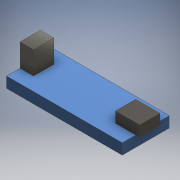
# Autodesk Inventor part: Arduino Nano
Saved by Autodesk Inventor 2016 (Build 200138000, 138)
## iProperties
Created: 2016-05-01
Part Number: Arduino Nano
Material: Generic
Document SubType Name: Modeling
Designer: Owner
Density: 1 g/cm^3
Appearance: Default
Author: Owner
Autodesk Inventor part; units mm, degrees
ref_plane "YZ Plane" through (0, 0, 0) normal (1, 0, 0) x (0, 1, 0)
ref_plane "XZ Plane" through (0, 0, 0) normal (0, 1, 0) x (-1, 0, 0)
ref_plane "XY Plane" through (0, 0, 0) normal (0, 0, 1) x (1, 0, 0)
sketch "Sketch1" plane through (0, 0, 0) normal (0, 0, 1) x (1, 0, 0)
  line L0 (0, 0) -> (43, 0)
  line L1 (43, 0) -> (43, 17.5)
  line L2 (43, 17.5) -> (0, 17.5)
  line L3 (0, 17.5) -> (0, 0)
  dimension "d0" = 43
  dimension "d1" = 17.5
  constraints: 8 end point, 2 parallel, 1 horizontal, 1 perpendicular
  measures "d0" distance of L0.start L0.end
  measures "d1" distance of L2.end L0.start
extrude "Extrusion1" add sketch "Sketch1" along normal blind 4
sketch "Sketch2" plane through (0, 0, 4) normal (0, 0, 1) x (1, 0, 0)
  line L0 (0, 0) -> (0, 5)
  line L1 (43, 17.5) -> (0, 17.5) projected
  line L2 (0, 17.5) -> (0, 12.5)
  line L3 (0, 17.5) -> (0, 0) projected
  line L4 (0, 12.5) -> (5, 12.5)
  line L5 (5, 12.5) -> (5, 5)
  line L6 (5, 5) -> (0, 5)
  line L7 (0, 12.5) -> (0, 5)
  line L8 (0.0001, 12.5) -> (0.0007, 5)
  dimension "d4" = 5
  dimension "d5" = 5
  dimension "d6" = 5
  constraints: 14 end point, 3 point on line, 2 perpendicular, 1 collinear, 1 horizontal, 1 vertical
  measures "d4" distance of L0.start L0.end
  measures "d5" distance of L1.end L2.end
  measures "d6" distance of L2.end L4.end
extrude "Extrusion2" add sketch "Sketch2" along normal blind 8.5
sketch "Sketch3" plane through (0, 0, 4) normal (0, 0, 1) x (1, 0, 0)
  line L0 (43, 0) -> (43, 17.5) projected
  line L1 (43, 0) -> (43, 5)
  line L2 (43, 5) -> (35.5, 5)
  line L3 (43, 17.5) -> (0, 17.5) projected
  line L4 (43, 17.5) -> (43, 12.5)
  line L5 (43, 12.5) -> (35.5, 12.5)
  line L6 (35.5, 12.5) -> (35.5, 5)
  point P0 (0, 0)
  dimension "d9" = 5
  dimension "d10" = 7.5
  dimension "d11" = 5
  constraints: 10 end point, 3 perpendicular, 2 point on line
  measures "d9" distance of L0.start L1.end
  measures "d10" distance of L1.end L2.end
  measures "d11" distance of L0.end L4.end
extrude "Extrusion3" add sketch "Sketch3" along normal blind 4
sketch "Sketch4" plane through (43, 0, 0) normal (1, 0, 0) x (0, 0, -1)
  line L0 (-8, 5) -> (-8, 12.5) projected
  line L1 (-4, 0) -> (-4, 5) projected
  line L2 (-8, 5) -> (-4, 5)
  line L3 (-4, 5) -> (-4, 12.5)
  line L4 (-4, 12.5) -> (-8, 12.5)
  line L5 (-8, 12.5) -> (-8, 5)
  point P0 (0, 0)
  constraints: 8 end point, 3 perpendicular, 1 horizontal
extrude "Extrusion4" add sketch "Sketch4" along normal blind 1.5
body "Solid1"
